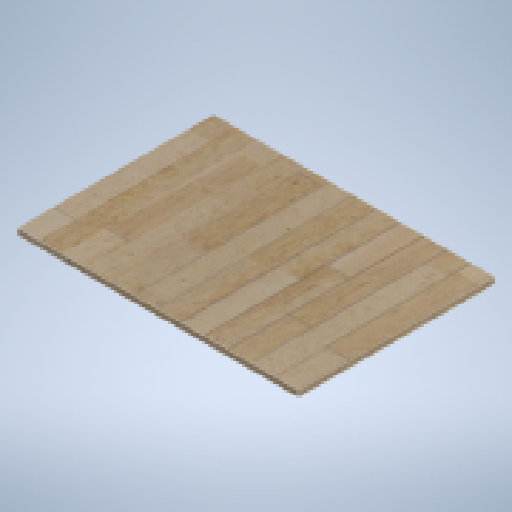
# Autodesk Inventor part: фанера1
Saved by Autodesk Inventor 2026.2 (Build 302298000, 298)
## iProperties
Created: 2026-05-20
Part Number: фанера1
Material: Wood (Maple)
Document SubType Name: Sheet Metal
Designer: admin
Density: 0.67 g/cm^3
Sheet Metal Rule: Default_mm
Appearance: Natural Maple - Glossy Dark Tint
Author: admin
Autodesk Inventor part; units mm, degrees
ref_plane "YZ Plane" through (0, 0, 0) normal (1, 0, 0) x (0, 1, 0)
ref_plane "XZ Plane" through (0, 0, 0) normal (0, 1, 0) x (-1, 0, 0)
ref_plane "XY Plane" through (0, 0, 0) normal (0, 0, 1) x (1, 0, 0)
sketch "Sketch1" plane through (0, 0, 0) normal (0, 1, 0) x (-1, 0, 0)
  line L0 (345, -237.5) -> (-345, -237.5)
  line L1 (-345, -237.5) -> (-345, 237.5)
  line L2 (-345, 237.5) -> (345, 237.5)
  line L3 (345, 237.5) -> (345, -237.5)
  line L4 (345, -237.5) -> (-345, 237.5) construction
  line L5 (-345, -237.5) -> (345, 237.5) construction
  point P0 (0, 0)
  dimension "d0" = 690
  dimension "d1" = 475
  measures "d0" distance of L1.end L2.end
  measures "d1" distance of L0.end L1.end
extrude "Plate1" add sketch "Sketch1" along normal blind 15
equation "\"d2\" = Thickness"
equation "\"BendRadius\" = Thickness"
equation "\"BendReliefWidth\" = Thickness"
equation "\"BendReliefDepth\" = 0.5 * Thickness"
equation "\"TransitionRadius\" = BendRadius"
equation "\"JacobiRadiusSize\" = BendRadius"
equation "\"GapSize\" = Thickness"
equation "\"Thickness\" = 15"
body "Solid1"
